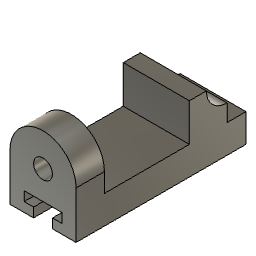
A2_AI22BTECH11005_2 (Autodesk Fusion 360 design; units mm, degrees)
Autodesk Fusion 360 part; units mm, degrees
sketch "Sketch1" plane through (0, 0, 0) normal (0, 1, 0) x (1, 0, 0)
  circle A0 centre (0, 0) radius 10
  line L0 (-35, 0) -> (-35, 50)
  line L1 (35, 50) -> (35, 0)
  arc A1 (-35, 0) -> (35, 0) centre (0, 0) ccw
  line L2 (-10, 50) -> (-10, 40)
  line L3 (-20, 40) -> (-10, 40)
  line L4 (-20, 40) -> (-20, 30)
  line L5 (20, 30) -> (20, 40)
  line L6 (20, 40) -> (10, 40)
  line L7 (10, 40) -> (10, 50)
  line L8 (-20, 30) -> (-18.0278, 30)
  line L9 (18.0278, 30) -> (20, 30)
  line L10 (-18.0278, 30) -> (18.0278, 30)
  line L11 (-35, 50) -> (-10, 50)
  line L12 (10, 50) -> (35, 50)
  dimension "d1" = 70
  dimension "d2" = 50
  dimension "d3" = 70
  dimension "d4" = 90
  dimension "d5" = 90
  constraint coincident A0.centre A1.centre
  constraint concentric A0 A1
  constraint tangent L0 A1
  constraint vertical L0
  constraint perpendicular L0 L11
  constraint tangent L1 A1
  constraint coincident L7.end L11
  constraint perpendicular L2 L3
  constraint perpendicular L3 L4
  constraint perpendicular L4 L8
  constraint perpendicular L5 L8
  constraint perpendicular L5 L6
  constraint collinear L11 L12
  measures "d1" diameter of A1
  measures "d2" distance of L0.start L0.end
  measures "d3" distance of L0.end L1.start
  measures "d4" angle of L1 L11
  measures "d5" angle of L0 L11
extrude "Extrude1" add sketch "Sketch1" along normal blind 30
sketch "Sketch2" plane through (0, 30, 0) normal (0, 1, 0) x (-1, 0, 0)
  circle A0 centre (0, 0) radius 10
  line L0 (20, -40) -> (10, -40)
  line L1 (10, -40) -> (10, -50)
  line L2 (10, -50) -> (35, -50)
  line L3 (35, -50) -> (35, 0)
  arc A1 (35, 0) -> (-35, 0) centre (0, 0) ccw
  line L4 (-35, 0) -> (-35, -50)
  line L5 (-35, -50) -> (-10, -50)
  line L6 (-10, -50) -> (-10, -40)
  line L7 (-10, -40) -> (-20, -40)
  line L8 (-20, -40) -> (-20, -30)
  line L9 (-20, -30) -> (20, -30)
  line L10 (20, -30) -> (20, -40)
  line L11 (-35, -50) -> (35, -50)
  line L12 (35, -50) -> (35, -20)
  line L13 (35, -20) -> (-35, -20)
  line L14 (-35, -20) -> (-35, -50)
  constraint coincident L4.end L5.start
  constraint coincident L2.end L3.start
  constraint coincident L3 L12.end
  constraint perpendicular L2 L12
  constraint coincident L4 L13.end
  constraint perpendicular L4 L13
  constraint perpendicular L5 L14
extrude "Extrude2" add sketch "Sketch2" along normal blind 90 contours L0 L1 L2 L3 L4 L5 L6 L7 L8 L9 L10 L11 L12 L13 L14 | L0 L1 L6 L7 L8 L9 L10 L11
sketch "Sketch3" plane through (0, 120, 0) normal (0, 1, 0) x (-1, 0, 0)
  line L0 (-35, -20) -> (-35, -50)
  line L1 (-35, -50) -> (35, -50)
  line L2 (35, -50) -> (35, -20)
  line L3 (35, -20) -> (-35, -20)
  line L4 (-35, -50) -> (35, -50)
  line L5 (35, -50) -> (35, 20)
  line L6 (35, 20) -> (-35, 20)
  line L7 (-35, 20) -> (-35, -50)
  dimension "d10" = 70
  dimension "d11" = 70
  constraint coincident L0.end L1.start
  constraint coincident L1.end L2.start
  constraint perpendicular L3 L5
  constraint perpendicular L5 L6
  measures "d10" distance of L1.end L5.end
  measures "d11" distance of L5.end L6.end
extrude "Extrude3" add sketch "Sketch3" along normal blind 18
sketch "Sketch4" plane through (-35, 0, 0) normal (-1, 0, 0) x (0, -1, 0)
  line L0 (0, -50) -> (0, 0)
  line L1 (0, 0) -> (-30, 0)
  line L2 (-30, 0) -> (-30, -20)
  line L3 (-30, -20) -> (-120, -20)
  line L4 (-120, -20) -> (-120, 20)
  line L5 (-120, 20) -> (-138, 20)
  line L6 (-138, 20) -> (-138, -50)
  line L7 (-138, -50) -> (0, -50)
  line L8 (-138, -50) -> (-160, -50)
  line L9 (-160, -50) -> (-160, -2)
  line L10 (-138, 20) -> (-138, -50)
  arc A0 (-160, -2) -> (-138, 20) centre (-160, 20) ccw
  dimension "d14" = 22
  constraint coincident L6.end L7.start
  constraint perpendicular L6 L8
  constraint perpendicular L8 L9
  constraint coincident L5.end L6.start
  measures "d14" distance of L6.end L8.end
extrude "Extrude4" add sketch "Sketch4" against normal blind 70 contours L6 L8 L9 L10 A0
sketch "Sketch5" plane through (0, 160, 0) normal (0, 1, 0) x (-1, 0, 0)
  line L0 (35, -50) -> (35, -2)
  line L1 (35, -2) -> (-35, -2)
  line L2 (-35, -2) -> (-35, -50)
  line L3 (-35, -50) -> (35, -50)
  line L4 (-35, -50) -> (35, -50)
  line L5 (35, -50) -> (35, -20)
  line L6 (35, -20) -> (-35, -20)
  line L7 (-35, -20) -> (-35, -50)
  dimension "d17" = 30
  constraint coincident L2.end L3.start
  constraint coincident L0.start L3.end
  constraint coincident L0 L5.end
  constraint coincident L2 L6.end
  constraint perpendicular L2 L6
  measures "d17" distance of L0.start L5.end
extrude "Extrude5" add sketch "Sketch5" along normal blind 20 contours L0 L2 L3 L4 L5 L6 L7
sketch "Sketch6" plane through (0, 0, 0) normal (0, -1, 0) x (1, 0, 0)
  circle A0 centre (0, 0) radius 10
  line L0 (-10, -40) -> (-20, -40)
  line L1 (-20, -40) -> (-20, -30)
  line L2 (-20, -30) -> (20, -30)
  line L3 (20, -30) -> (20, -40)
  line L4 (20, -40) -> (10, -40)
  line L5 (10, -40) -> (10, -50)
  line L6 (10, -50) -> (35, -50)
  line L7 (35, -50) -> (35, 0)
  arc A1 (35, 0) -> (-35, 0) centre (0, 0) ccw
  line L8 (-35, 0) -> (-35, -50)
  line L9 (-35, -50) -> (-10, -50)
  line L10 (-10, -50) -> (-10, -40)
  line L11 (-10, -50) -> (-10, -40)
  line L12 (-10, -40) -> (-20, -40)
  line L13 (-20, -40) -> (-20, -30)
  line L14 (-20, -30) -> (20, -30)
  line L15 (20, -30) -> (20, -40)
  line L16 (20, -40) -> (10, -40)
  line L17 (10, -40) -> (10, -50)
  line L18 (-10, -50) -> (10, -50)
  constraint coincident L9.end L10.start
  constraint coincident L0.start L10.end
  constraint coincident L0.end L1.start
  constraint coincident L1.end L2.start
  constraint coincident L2.end L3.start
  constraint coincident L3.end L4.start
  constraint coincident L4.end L5.start
  constraint coincident L5.end L6.start
extrude "Extrude6" cut sketch "Sketch6" against normal blind 210 contours L0 L1 L2 L3 L4 L5 L10 L11 L12 L13 L14 L15 L16 L17 L18
